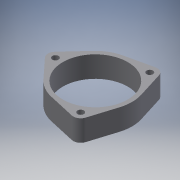
# Autodesk Inventor part: Chamber Holder
Saved by Autodesk Inventor 2018.1 (Build 221171000, 171)
## iProperties
Created: 2024-06-08
Part Number: Chamber Holder
Material: Generic
Document SubType Name: Modeling
Designer: Enrico
Density: 1 g/cm^3
Appearance: Default
Author: Enrico
Autodesk Inventor part; units mm, degrees
ref_plane "YZ Plane" through (0, 0, 0) normal (1, 0, 0) x (0, 1, 0)
ref_plane "XZ Plane" through (0, 0, 0) normal (0, 1, 0) x (-1, 0, 0)
ref_plane "XY Plane" through (0, 0, 0) normal (0, 0, 1) x (1, 0, 0)
sketch "Sketch1" plane through (0, 0, 0) normal (0, 0, 1) x (1, 0, 0)
  circle A0 centre (130.9, -80) radius 15 construction
  line L0 (0, 0) -> (117.2543, 0) construction
  line L1 (-60.9, -65.8) -> (60.9, -65.8) projected
  line L2 (60.9, -94.2) -> (60.9, -65.8) projected
  line L3 (60.9, -94.2) -> (-60.9, -94.2) projected
  line L4 (-60.9, -65.8) -> (-60.9, -94.2) projected
  circle A1 centre (130.9, -80) radius 15.3
  circle A2 centre (130.9, -80) radius 17.3
  circle A3 centre (112.1, -80) radius 1.5
  circle A4 centre (112.1, -80) radius 3.5
  line L5 (109.5309, -77.6231) -> (118.2011, -68.2515)
  line L6 (109.5309, -82.3769) -> (118.2011, -91.7485)
  circle A5 centre (-45.9, -80) radius 3.15 projected
  circle A6 centre (45.9, -80) radius 3.15 projected
  point P0 (60.9, -80)
  dimension "d0" = 30
  dimension "d1" = 70
  dimension "d2" = 0.3
  dimension "d3" = 2
  dimension "d4" = 3
  dimension "d6" = 2
  constraints: 6 end point, 5 centre point, 5 tangent, 4 point on circle, 2 horizontal alignment, 1 horizontal, 1 midpoint
  measures "d0" diameter of A0
  measures "d1" distance from line of L2 A0.centre
  measures "d2" radial gap between concentric circles of A0 A1
  measures "d3" radial gap between concentric circles of A1 A2
  measures "d4" diameter of A3
  measures "d6" radial gap between concentric circles of A3 A4
extrude "Extrusion1" add sketch "Sketch1" against normal blind 10 contours A4 A2 | A4 A2 | A4 L5 A2 | A2 A4 | A2 L6 A4
pattern_circular "Circular Pattern1" count 3 over 360 about axis through (130.9, -80, 0) along (0, 0, -1) of "Extrusion1"
body "Solid1"
